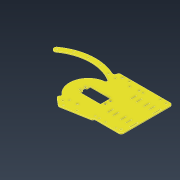
# Autodesk Inventor part: wstepna_geometria_wersja_2
Saved by Autodesk Inventor 2022 (Build 260153000, 153)
## iProperties
Created: 2022-02-09
Part Number: wstepna_geometria_wersja_2
Material: Generic
Document SubType Name: Modeling
Designer: Tomasz Krakowski
Density: 1 g/cm^3
Appearance: Kanarkowa
Mass: 25.2721 g
Surface Area: 279.808 cm^2
Volume: 25.2721 cm^3
Author: Tomasz Krakowski
Autodesk Inventor part; units mm, degrees
ref_plane "YZ Plane" through (0, 0, 0) normal (1, 0, 0) x (0, 1, 0)
ref_plane "XZ Plane" through (0, 0, 0) normal (0, 1, 0) x (-1, 0, 0)
ref_plane "XY Plane" through (0, 0, 0) normal (0, 0, 1) x (1, 0, 0)
sketch "Sketch1" plane through (0, 0, 0) normal (0, 1, 0) x (-1, 0, 0)
  arc A0 (-0.3814, 2.9757) -> (-3, 0) centre (0, 0) ccw
  line L0 (-35, 45.25) -> (5, 45.25)
  line L1 (5, 45.25) -> (5, 24.75)
  line L2 (5, 24.75) -> (-35, 24.75)
  line L3 (-35, 24.75) -> (-35, 45.25)
  line L4 (-35, 45.25) -> (5, 24.75) construction
  line L5 (5, 45.25) -> (-35, 24.75) construction
  line L6 (-5, 35) -> (-15, 35) construction
  circle A1 centre (9.25, 30) radius 2.1
  circle A2 centre (9.25, 40) radius 2.1
  line L7 (9.25, 40) -> (9.25, 30) construction
  circle A3 centre (-39.25, 40) radius 2.1
  circle A4 centre (-39.25, 30) radius 2.1
  line L8 (-39.25, 40) -> (-39.25, 30) construction
  line L9 (-39.25, 35) -> (-15, 35) construction
  line L10 (-5, 35) -> (9.25, 35) construction
  line L11 (-39.25, 40) -> (9.25, 40) construction
  line L12 (-39.25, 30) -> (9.25, 30) construction
  line L13 (-15, 35) -> (-15, 40) construction
  circle A5 centre (-5, 35) radius 10 construction
  circle A6 centre (-24.5, 35) radius 10 construction
  arc A7 (-0.3814, 2.9757) -> (0, 75) centre (-5, 39.0133) ccw
  line L14 (-105, 0) -> (0, 0) construction
  line L15 (-3, 0) -> (-105, 0) construction
  arc A8 (-3, 0) -> (-0.3814, -2.9757) centre (0, 0) ccw
  arc A9 (-1.6619, -2.4976) -> (97.0992, -0.9275) centre (46.5785, 70) ccw
  arc A10 (102.9008, -9.0725) -> (97.0992, -0.9275) centre (100, -5) ccw
  line L16 (0, 0) -> (100, 0) construction
  arc A11 (5.6849, -18.0476) -> (102.9008, -9.0725) centre (46.5785, 70) ccw
  line L17 (0, 75) -> (0, 0) construction
  line L18 (0, 0) -> (0, -15.1769) construction
  line L19 (0, 0) -> (-105, 0) construction
  line L20 (0, 75) -> (-105, 75)
  line L21 (-105, 75) -> (-105, -25)
  line L22 (0, -21.6754) -> (0, -21)
  line L23 (-4, -25) -> (-105, -25)
  arc A12 (5.6849, -18.0476) -> (0, -21.6754) centre (4, -21.6754) ccw
  arc A13 (-4, -25) -> (0, -21) centre (-4, -21) ccw
  point P0 (-5, -39.0133)
  point P1 (0, -25)
  dimension "d0" = 6
  dimension "d1" = 40
  dimension "d2" = 20.5
  dimension "d4" = 48.5
  dimension "d5" = 4.2
  dimension "d6" = 10
  dimension "d11" = 10.5
  dimension "d13" = 5
  dimension "d47" = 10
  dimension "d48" = 100
  dimension "d49" = 100
  dimension "d60" = 14.25
  dimension "d68" = 70
  dimension "d71" = 0
  dimension "d73" = 25
  dimension "d75" = 105
  dimension "d76" = 4
  dimension "d77" = 4
  dimension "d108" = 75
  dimension "d109" = 35
  dimension "d110" = 5
  constraints: 48 end point, 18 point on circle, 14 centre point, 10 tangent, 7 horizontal, 7 point on line, 5 midpoint, 5 perpendicular, 4 coincident, 4 equal radius, 3 collinear, 3 vertical, 2 parallel, 2 symmetric about line, 1 other
  measures "d0" diameter of A0
  measures "d1" distance between parallel lines of L3 L1
  measures "d2" distance between parallel lines of L0 L2
  measures "d4" distance between parallel lines of L8 L7
  measures "d5" diameter of A1
  measures "d6" distance of L7.end L7.start
  measures "d11" distance from line of L3 A6.centre
  measures "d13" horizontal distance of point (0, 0) A7.centre
  measures "d47" diameter of A10
  measures "d48" distance of L16.end point (0, 0)
  measures "d49" horizontal distance of point (0, 0) A10.centre
  measures "d60" distance from line of A5.centre L7
  measures "d68" vertical distance of point (0, 0) A9.centre
  measures "d71" distance between parallel lines of L19 L15
  measures "d73" distance from line of L23 point (0, 0)
  measures "d75" horizontal distance of point (0, 0) L20.end
  measures "d76" radius of A12
  measures "d77" radius of A13
  measures "d108" distance from line of point (0, 0) L20
  measures "d109" distance from line of L6 L14.end
  measures "d110" horizontal distance of A0.centre L6.start
extrude "Extrusion1" add sketch "Sketch1" along normal blind 2
sketch "Szkic5" plane through (0, 2, 0) normal (0, 1, 0) x (1, 0, 0)
  circle A0 centre (12.5, 20) radius 2.1
  circle A1 centre (97.5, 20) radius 2.1
  circle A2 centre (12.5, -67.5) radius 2.1
  circle A3 centre (97.5, -67.5) radius 2.1
  line L0 (12.5, 20) -> (97.5, 20) construction
  line L1 (97.5, -67.5) -> (97.5, 20) construction
  line L2 (12.5, -67.5) -> (97.5, -67.5) construction
  line L3 (0, -75) -> (105, -75) construction
  line L4 (105, -75) -> (105, 25) construction
  line L5 (105, 25) -> (4, 25) construction
  line L6 (0, 21) -> (0, 21.6754) construction
  point P0 (0, 0)
  dimension "d84" = 7.5
  dimension "d85" = 7.5
  dimension "d88" = 4.2
  dimension "d89" = 85
  dimension "d112" = 85
  dimension "d153" = 87.5
  constraints: 6 end point, 4 centre point, 3 equal radius, 2 horizontal, 1 vertical
  measures "d84" distance between parallel lines of L3 L2
  measures "d85" distance between parallel lines of L4 L1
  measures "d88" diameter of A0
  measures "d89" distance of L2.start L1.start
  measures "d112" distance of L0.start L0.end
  measures "d153" distance between parallel lines of L2 L0
extrude "Wyciągnięcie proste4" cut sketch "Szkic5" against normal up to surface (2 mm away)
sketch "Szkic6" plane through (0, 2, 0) normal (0, 1, 0) x (1, 0, 0)
  line L0 (103, -55) -> (100.9, -55)
  line L1 (100.9, -55) -> (100.9, -40)
  line L2 (100.9, -40) -> (103, -40)
  line L3 (103, -40) -> (103, -55)
  line L4 (103, -10) -> (100.9, -10)
  line L5 (100.9, -10) -> (100.9, 5)
  line L6 (100.9, 5) -> (103, 5)
  line L7 (103, 5) -> (103, -10)
  line L8 (105, 25) -> (4, 25) construction
  line L9 (100.9, -40) -> (100.9, -10) construction
  line L10 (105, -75) -> (105, 25) construction
  line L11 (100.9, -25) -> (105, -25) construction
  point P0 (0, 0)
  dimension "d92" = 15
  dimension "d94" = 30
  dimension "d168" = 2.1
  dimension "d169" = 2
  constraints: 20 end point, 4 parallel, 3 perpendicular, 2 collinear, 2 horizontal, 1 midpoint, 1 point on line, 1 vertical, 2 other
  measures "d92" distance of L4.end L5.end
  measures "d94" distance between parallel lines of L4 L2
  measures "d168" distance between parallel lines of L7 L5
extrude "Wyciągnięcie proste5" cut sketch "Szkic6" against normal up to surface (2 mm away)
sketch "Sketch7" plane through (0, 2, 0) normal (0, 1, 0) x (1, 0, 0)
  circle A0 centre (50, -70) radius 1.6
  circle A1 centre (57.5, -70) radius 1.6
  line L0 (50, -70) -> (57.5, -70) construction
  line L1 (105, -75) -> (105, 25) construction
  line L2 (0, -75) -> (105, -75) construction
  circle A2 centre (50, 15) radius 1.6
  circle A3 centre (57.5, 15) radius 1.6
  line L3 (50, 15) -> (57.5, 15) construction
  line L4 (50, 15) -> (50, -70) construction
  line L5 (57.5, 15) -> (57.5, -70) construction
  line L6 (105, 25) -> (4, 25) construction
  point P0 (0, 0)
  point P1 (105, -55)
  dimension "d98" = 3.2
  dimension "d100" = 7.5
  dimension "d101" = 5
  dimension "d104" = 3.2
  dimension "d152" = 85
  dimension "d167" = 50
  constraints: 8 end point, 4 centre point, 2 equal radius, 2 horizontal, 2 perpendicular
  measures "d98" diameter of A0
  measures "d100" distance of L0.start L0.end
  measures "d101" distance between parallel lines of L0 L2
  measures "d104" diameter of A2
  measures "d152" distance between parallel lines of L3 L0
  measures "d167" distance from line of L4 point (0, 0)
extrude "Extrusion6" cut sketch "Sketch7" against normal up to next
sketch "Sketch9" plane through (0, 0, 0) normal (0, -1, 0) x (1, 0, 0)
  line L0 (0, 75) -> (105, 75) construction
  line L1 (7.5, 75) -> (-3.7488, 88.4058)
  line L2 (-3.7488, 88.4058) -> (-20.9848, 73.9431)
  line L3 (-20.9848, 73.9431) -> (-16.3455, 68.4142)
  arc A0 (0, 75) -> (0.3814, 2.9757) centre (5, 39.0133) ccw construction
  arc A1 (0, 75) -> (-16.3455, 68.4142) centre (5, 39.0133) ccw
  line L4 (0, 75) -> (7.5, 75)
  point P0 (0, 0)
  dimension "d126" = 22.5
  dimension "d128" = 17.5
  dimension "d129" = 130
  dimension "d166" = 7.5
  constraints: 8 end point, 3 point on circle, 2 perpendicular, 1 centre point, 1 coincident, 1 horizontal, 1 point on line
  measures "d126" distance between parallel lines of L1 L3
  measures "d128" distance from line of L1.start L2
  measures "d129" angle of L0 L1
  measures "d166" horizontal distance of L1.start point (0, 0)
extrude "Extrusion7" add sketch "Sketch9" against normal up to surface (2 mm away)
sketch "Sketch8" plane through (0, 2, 0) normal (0, 1, 0) x (1, 0, 0)
  line L0 (-1.8203, -68.6056) -> (-7.6054, -75.5) construction
  line L1 (0, -75) -> (105, -75) construction
  circle A0 centre (12.5, -67.5) radius 2.1 construction
  line L2 (-7.6054, -75.5) -> (12.5, -75.5) construction
  line L3 (12.5, -75.5) -> (12.5, -67.5) construction
  line L4 (-7.6054, -75.5) -> (-12.3668, -81.1744) construction
  line L5 (-3.7488, -88.4058) -> (-20.9848, -73.9431) construction
  line L6 (-3.7488, -88.4058) -> (-20.9848, -73.9431) construction
  point P0 (0, 0)
  dimension "d114" = 9
  dimension "d115" = 50
  dimension "d132" = 22.5
  dimension "d133" = 11.25
  dimension "d134" = 8
  constraints: 8 end point, 2 coincident, 2 perpendicular, 1 horizontal, 1 midpoint
  measures "d114" distance of L0.start L0.end
  measures "d115" angle of L2 L0
  measures "d132" distance of L5.start L5.end
  measures "d133" distance of L5.start L4.end
  measures "d134" distance from line of L3.end L2
hole "Hole1" at (-1.8203, 2, 68.6056) at (-7.6054, 2, 75.5) direction (0, -1, 0) diameter 3.2 depth 7.5
sketch "Sketch11" plane through (0, 2, 0) normal (0, 1, 0) x (1, 0, 0)
  line L0 (-3.7488, -88.4058) -> (-20.9848, -73.9431) construction
  line L1 (-3.7488, -88.4058) -> (52.5, -78.4876)
  line L2 (7.5, -75) -> (105, -75) construction
  line L3 (7.5, -75) -> (-3.7488, -88.4058)
  line L4 (7.5, -75) -> (52.5, -75)
  line L5 (52.5, -78.4876) -> (52.5, -75)
  point P0 (0, 0)
  dimension "d149" = 100
  dimension "d150" = 45
  constraints: 8 end point, 1 perpendicular, 1 point on line
  measures "d149" angle of L1 L5
  measures "d150" distance from line of L2.start L5
extrude "Extrusion8" add sketch "Sketch11" against normal up to surface (2 mm away)
fillet "Fillet2" radius 3 5 edges at (52.5, 1, 75) (52.5, 1, 78.4876) (-3.7488, 1, 88.4058) (-20.9848, 1, 73.9431) (-16.3455, 1, 68.4142)
sketch "Szkic12" plane through (0, 2, 0) normal (0, 1, 0) x (1, 0, 0)
  line L0 (6, 12.5) -> (34, 12.5) construction
  circle A0 centre (6, 12.5) radius 1.5
  circle A1 centre (34, 12.5) radius 1.5
  line L1 (105, 25) -> (4, 25) construction
  point P0 (0, 0)
  dimension "d154" = 3
  dimension "d155" = 12.5
  dimension "d156" = 6
  dimension "d157" = 28
  constraints: 2 centre point, 2 coincident, 2 end point, 1 equal radius, 1 horizontal
  measures "d154" diameter of A0
  measures "d155" distance between parallel lines of L1 L0
  measures "d156" horizontal distance of L0.start point (0, 0)
  measures "d157" distance of L0.start L0.end
extrude "Wyciągnięcie proste9" cut sketch "Szkic12" against normal up to surface (2 mm away)
fillet "Fillet3" radius 5 2 edges at (105, 1, 75) (105, 1, -25)
sketch "Sketch13" plane through (0, 0, 0) normal (0, -1, 0) x (1, 0, 0)
  line L0 (-8, 32) -> (-5, 32)
  line L1 (-5, 32) -> (-5, 38)
  line L2 (-5, 38) -> (-8, 38)
  line L3 (-8, 38) -> (-8, 32)
  line L4 (-8, 32) -> (-5, 38) construction
  line L5 (-5, 32) -> (-8, 38) construction
  line L6 (-5, 24.75) -> (-5, 45.25) construction
  line L7 (-5, 45.25) -> (-5, 24.75) construction
  line L8 (-5, 35) -> (-6.5, 35) construction
  point P0 (0, 0)
  dimension "d161" = 3
  dimension "d162" = 6
  constraints: 14 end point, 3 midpoint, 2 parallel, 2 perpendicular, 1 collinear, 1 horizontal
  measures "d161" distance from line of L8.start L3
  measures "d162" distance between parallel lines of L2 L0
extrude "Extrusion10" cut sketch "Sketch13" against normal through all
fillet "Fillet4" radius 2 4 edges at (-5, 1, 32) (-5, 1, 38) (-8, 1, 32) (-8, 1, 38)
sketch "Sketch14" plane through (0, 2, 0) normal (0, 1, 0) x (1, 0, 0)
  arc A0 (1.6619, 2.4976) -> (-97.0992, 0.9275) centre (-46.5785, -70) ccw construction
  arc A1 (-102.9008, 9.0725) -> (-97.0992, 0.9275) centre (-100, 5) ccw construction
  arc A2 (13.245, 0) -> (-100, 5) centre (-46.5785, -70) ccw construction
  arc A3 (0.3814, -2.9757) -> (1.6619, 2.4976) centre (0, 0) ccw construction
  line L0 (0, 0) -> (13.245, 0) construction
  line L1 (0.6999, -82.5442) -> (45.0162, -74.7301) construction
  line L2 (-2.3711, -88.1629) -> (50.3991, -78.858) construction
  line L3 (0.6999, -82.5442) -> (1.5681, -87.4683) construction
  line L4 (70, -70) -> (90, -70) construction
  line L5 (55.5, -75) -> (100, -75) construction
  line L6 (25, 21) -> (85, 21) construction
  line L7 (100, 25) -> (4, 25) construction
  circle A4 centre (12.5, 20) radius 2.1 construction
  point P0 (-78.7683, 16.2709)
  point P1 (-78.7683, 16.2709)
  point P2 (-55.3429, 21.6626)
  point P3 (-55.3429, 21.6626)
  point P4 (-31.3202, 20.8077)
  point P5 (-31.3202, 20.8077)
  point P6 (-8.3374, 13.7643)
  point P7 (-8.3374, 13.7643)
  point P8 (22.8581, -78.6371)
  dimension "d172" = 60
  dimension "d174" = 5
  dimension "d175" = 45
  dimension "d176" = 4
  dimension "d177" = 5
  dimension "d178" = 20
  dimension "d179" = 10
  dimension "d180" = 4
  dimension "d181" = 60
  dimension "d182" = 12.5
  constraints: 10 coincident, 10 end point, 3 horizontal, 2 point on circle, 1 centre point, 1 midpoint, 13 other
  measures "d175" distance of L1.end L1.start
  measures "d176" distance from line of point (-2.371, -88.163) L3
  measures "d177" distance between parallel lines of L5 L4
  measures "d178" distance of L4.start L4.end
  measures "d179" horizontal distance of L5.end L4.end
  measures "d180" distance between parallel lines of L7 L6
  measures "d181" distance of L6.end L6.start
  measures "d182" horizontal distance of L6.start A4.centre
hole "Hole3" at (-100, 2, -5) at (-78.7683, 2, -16.2709) at (-55.3429, 2, -21.6626) at (-31.3202, 2, -20.8077) at (-8.3374, 2, -13.7643) at (25, 2, -21) at (85, 2, -21) at (0.6999, 2, 82.5442) at (22.8581, 2, 78.6371) at (70, 2, 70) at (90, 2, 70) direction (0, -1, 0) diameter 3.2 end through all
sketch "Sketch15" plane through (0, 2, 0) normal (0, 1, 0) x (1, 0, 0)
  line L0 (65.5, 4) -> (67, 4)
  line L1 (67, 4) -> (67, -7)
  line L2 (67, -7) -> (65.5, -7)
  line L3 (65.5, -7) -> (65.5, 4)
  line L4 (55, 4) -> (56.5, 4)
  line L5 (56.5, 4) -> (56.5, -7)
  line L6 (56.5, -7) -> (55, -7)
  line L7 (55, -7) -> (55, 4)
  line L8 (65.5, -41) -> (67, -41)
  line L9 (67, -41) -> (67, -52)
  line L10 (67, -52) -> (65.5, -52)
  line L11 (65.5, -52) -> (65.5, -41)
  line L12 (55, -41) -> (56.5, -41)
  line L13 (56.5, -41) -> (56.5, -52)
  line L14 (56.5, -52) -> (55, -52)
  line L15 (55, -52) -> (55, -41)
  line L16 (90.5, 4) -> (92, 4)
  line L17 (92, 4) -> (92, -7)
  line L18 (92, -7) -> (90.5, -7)
  line L19 (90.5, -7) -> (90.5, 4)
  line L20 (80, 4) -> (81.5, 4)
  line L21 (81.5, 4) -> (81.5, -7)
  line L22 (81.5, -7) -> (80, -7)
  line L23 (80, -7) -> (80, 4)
  line L24 (90.5, -41) -> (92, -41)
  line L25 (92, -41) -> (92, -52)
  line L26 (92, -52) -> (90.5, -52)
  line L27 (90.5, -52) -> (90.5, -41)
  line L28 (80, -41) -> (81.5, -41)
  line L29 (81.5, -41) -> (81.5, -52)
  line L30 (81.5, -52) -> (80, -52)
  line L31 (80, -52) -> (80, -41)
  point P0 (0, 0)
  dimension "d190" = 1.5
  dimension "d191" = 11
  dimension "d192" = 9
  dimension "d193" = 55
  dimension "d194" = 4
  dimension "d197" = 45
  dimension "d200" = 25
  constraints: 64 end point, 8 point on line, 4 parallel, 3 collinear, 3 horizontal, 2 perpendicular, 1 vertical, 46 other
  measures "d190" distance of L0.end L0.start
  measures "d191" distance of L2.end L0.start
  measures "d192" distance between parallel lines of L3 L5
  measures "d193" distance from line of L7 point (0, 0)
  measures "d194" vertical distance of L4.start point (0, 0)
  measures "d197" distance of L0.start L8.start
  measures "d200" distance of L0.start L16.start
extrude "Extrusion11" cut sketch "Sketch15" against normal through all
sketch "Sketch16" plane through (0, 2, 0) normal (0, 1, 0) x (1, 0, 0)
  line L0 (81.5, -41) -> (81.5, -52) projected
  line L1 (81.5, -52) -> (80, -52) projected
  line L2 (80, -52) -> (80, -41) projected
  line L3 (80, -41) -> (81.5, -41) projected
  line L4 (81.5, 4) -> (81.5, -7) projected
  line L5 (81.5, -7) -> (80, -7) projected
  line L6 (80, -7) -> (80, 4) projected
  line L7 (80, 4) -> (81.5, 4) projected
  line L8 (67, 4) -> (67, -7) projected
  line L9 (67, -7) -> (65.5, -7) projected
  line L10 (65.5, -7) -> (65.5, 4) projected
  line L11 (65.5, 4) -> (67, 4) projected
  line L12 (67, -41) -> (67, -52) projected
  line L13 (67, -52) -> (65.5, -52) projected
  line L14 (65.5, -52) -> (65.5, -41) projected
  line L15 (65.5, -41) -> (67, -41) projected
  line L16 (92, -41) -> (92, -52) projected
  line L17 (92, -52) -> (90.5, -52) projected
  line L18 (90.5, -52) -> (90.5, -41) projected
  line L19 (90.5, -41) -> (92, -41) projected
  line L20 (92, 4) -> (92, -7) projected
  line L21 (92, -7) -> (90.5, -7) projected
  line L22 (90.5, -7) -> (90.5, 4) projected
  line L23 (90.5, 4) -> (92, 4) projected
  line L24 (56.5, 4) -> (56.5, -7) projected
  line L25 (56.5, -7) -> (55, -7) projected
  line L26 (55, -7) -> (55, 4) projected
  line L27 (55, 4) -> (56.5, 4) projected
  line L28 (56.5, -41) -> (56.5, -52) projected
  line L29 (56.5, -52) -> (55, -52) projected
  line L30 (55, -52) -> (55, -41) projected
  line L31 (55, -41) -> (56.5, -41) projected
  circle A0 centre (70, -70) radius 1.6 projected
  circle A1 centre (0.6999, -82.5442) radius 1.6 projected
  circle A2 centre (25, 21) radius 1.6 projected
  circle A3 centre (-31.3202, 20.8077) radius 1.6 projected
  circle A4 centre (-78.7683, 16.2709) radius 1.6 projected
  circle A5 centre (-100, 5) radius 1.6 projected
  circle A6 centre (-55.3429, 21.6626) radius 1.6 projected
  circle A7 centre (-8.3374, 13.7643) radius 1.6 projected
  circle A8 centre (85, 21) radius 1.6 projected
  circle A9 centre (22.8581, -78.6371) radius 1.6 projected
  circle A10 centre (90, -70) radius 1.6 projected
  line L32 (-8, -36.127) -> (-8, -33.873) projected
  arc A11 (-6.5, -31.9365) -> (-8, -33.873) centre (-6, -33.873) ccw projected
  arc A12 (-6.5, -31.9365) -> (-5, -30) centre (-7, -30) ccw projected
  line L33 (-5, -30) -> (-5, -24.75) projected
  line L34 (-5, -24.75) -> (35, -24.75) projected
  line L35 (35, -24.75) -> (35, -45.25) projected
  line L36 (35, -45.25) -> (-5, -45.25) projected
  line L37 (-5, -45.25) -> (-5, -40) projected
  arc A13 (-5, -40) -> (-6.5, -38.0635) centre (-7, -40) ccw projected
  arc A14 (-8, -36.127) -> (-6.5, -38.0635) centre (-6, -36.127) ccw projected
  arc A15 (105, 20) -> (100, 25) centre (100, 20) ccw projected
  line L38 (100, 25) -> (4, 25) projected
  arc A16 (4, 25) -> (0, 21) centre (4, 21) ccw projected
  line L39 (0, 21) -> (0, 21.6754) projected
  arc A17 (-5.6849, 18.0476) -> (0, 21.6754) centre (-4, 21.6754) ccw projected
  arc A18 (-5.6849, 18.0476) -> (-102.9008, 9.0725) centre (-46.5785, -70) ccw projected
  arc A19 (-102.9008, 9.0725) -> (-97.0992, 0.9275) centre (-100, 5) ccw projected
  arc A20 (1.6619, 2.4976) -> (-97.0992, 0.9275) centre (-46.5785, -70) ccw projected
  arc A21 (0.3814, -2.9757) -> (1.6619, 2.4976) centre (0, 0) ccw projected
  arc A22 (0.3814, -2.9757) -> (-18.6731, -66.5747) centre (5, -39.0133) ccw projected
  arc A23 (-18.3296, -70.7788) -> (-18.6731, -66.5747) centre (-20.6278, -68.8504) ccw projected
  line L40 (-19.0564, -71.6449) -> (-18.3296, -70.7788) projected
  arc A24 (-19.0564, -71.6449) -> (-18.6866, -75.8714) centre (-16.7583, -73.5733) ccw projected
  line L41 (-4.8204, -87.5066) -> (-18.6866, -75.8714) projected
  arc A25 (-4.8204, -87.5066) -> (-2.3711, -88.1629) centre (-2.8921, -85.2084) ccw projected
  line L42 (-2.3711, -88.1629) -> (50.3991, -78.858) projected
  arc A26 (50.3991, -78.858) -> (52.6891, -76.9518) centre (49.8781, -75.9036) ccw projected
  arc A27 (55.5, -75) -> (52.6891, -76.9518) centre (55.5, -78) ccw projected
  line L43 (55.5, -75) -> (100, -75) projected
  arc A28 (100, -75) -> (105, -70) centre (100, -70) ccw projected
  line L44 (105, -70) -> (105, 20) projected
  circle A29 centre (6, 12.5) radius 1.5 projected
  circle A30 centre (34, 12.5) radius 1.5 projected
  circle A31 centre (-1.8203, -68.6056) radius 1.6 projected
  circle A32 centre (-7.6054, -75.5) radius 1.6 projected
  circle A33 centre (50, 15) radius 1.6 projected
  circle A34 centre (50, -70) radius 1.6 projected
  circle A35 centre (57.5, -70) radius 1.6 projected
  circle A36 centre (57.5, 15) radius 1.6 projected
  line L45 (103, -55) -> (100.9, -55) projected
  line L46 (100.9, -55) -> (100.9, -40) projected
  line L47 (100.9, -40) -> (103, -40) projected
  line L48 (103, -40) -> (103, -55) projected
  line L49 (100.9, -10) -> (100.9, 5) projected
  line L50 (100.9, 5) -> (103, 5) projected
  line L51 (103, 5) -> (103, -10) projected
  line L52 (103, -10) -> (100.9, -10) projected
  circle A37 centre (12.5, -67.5) radius 2.1 projected
  circle A38 centre (97.5, -67.5) radius 2.1 projected
  circle A39 centre (97.5, 20) radius 2.1 projected
  circle A40 centre (12.5, 20) radius 2.1 projected
  circle A41 centre (39.25, -30) radius 2.1 projected
  circle A42 centre (39.25, -40) radius 2.1 projected
  circle A43 centre (-9.25, -40) radius 2.1 projected
  circle A44 centre (-9.25, -30) radius 2.1 projected
  circle A45 centre (16, 7.5) radius 6
  circle A46 centre (30, 0.5) radius 6
  circle A47 centre (44, 7.5) radius 6
  line L53 (30, 0.5) -> (30, -5.5) construction
  circle A48 centre (16, -7.5) radius 6
  circle A49 centre (30, -14.5) radius 6
  circle A50 centre (44, -7.5) radius 6
  circle A51 centre (66, 12.5) radius 6
  circle A52 centre (80, 12.5) radius 6
  circle A53 centre (92.5, 12.5) radius 4
  line L54 (80, 12.5) -> (92.5, 12.5) construction
  line L55 (66, 12.5) -> (80, 12.5) construction
  circle A54 centre (54.5, -17) radius 6
  circle A55 centre (68.5, -17) radius 6
  circle A56 centre (82.5, -17) radius 6
  circle A57 centre (96.5, -17) radius 6
  circle A58 centre (54.5, -31) radius 6
  circle A59 centre (68.5, -31) radius 6
  circle A60 centre (82.5, -31) radius 6
  circle A61 centre (96.5, -31) radius 6
  line L56 (96.5, -17) -> (96.5, -31) construction
  line L57 (90.5, -41) -> (92, -41) construction
  line L58 (90.5, -7) -> (90.5, -41) construction
  line L59 (96.5, -24) -> (90.5, -24) construction
  arc A62 (0.3814, -2.9757) -> (-18.6731, -66.5747) centre (5, -39.0133) ccw construction
  circle A63 centre (5, -39.0133) radius 26.5 construction
  circle A64 centre (0.3983, -12.9159) radius 6
  circle A65 centre (-15.3002, -21.9794) radius 6
  circle A66 centre (-21.5, -39.0133) radius 6
  circle A67 centre (-15.3002, -56.0472) radius 6
  line L60 (5, -39.0133) -> (0.3983, -12.9159) construction
  line L61 (5, -39.0133) -> (31.5, -39.0133) construction
  circle A68 centre (-1.3002, -56.0472) radius 6
  line L62 (-15.3002, -56.0472) -> (-1.3002, -56.0472) construction
  circle A69 centre (12.6998, -56.0472) radius 6
  circle A70 centre (26.6998, -56.0472) radius 6
  circle A71 centre (40.6998, -56.0472) radius 6
  circle A72 centre (33.6998, -69.0472) radius 6
  line L63 (26.6998, -56.0472) -> (40.6998, -56.0472) construction
  line L64 (33.6998, -69.0472) -> (33.6998, -56.0472) construction
  circle A73 centre (54.5, -59.5) radius 6
  line L65 (54.5, -59.5) -> (54.5, -31) construction
  circle A74 centre (68.5, -59.5) radius 6
  circle A75 centre (82.5, -59.5) radius 6
  point P0 (34, -2.5)
  point P1 (30, -20.5)
  dimension "d205" = 12
  dimension "d206" = 14
  dimension "d207" = 14
  dimension "d208" = 7
  dimension "d209" = 7
  dimension "d212" = 15
  dimension "d217" = 16
  dimension "d218" = 7.5
  dimension "d219" = 12
  dimension "d222" = 14
  dimension "d227" = 12.5
  dimension "d228" = 8
  dimension "d229" = 66
  dimension "d230" = 12.5
  dimension "d233" = 14
  dimension "d236" = 14
  dimension "d239" = 6
  dimension "d242" = 120
  dimension "d244" = 53
  dimension "d245" = 100
  dimension "d246" = 14
  dimension "d249" = 14
  dimension "d254" = 13
  dimension "d256" = 28.5
  dimension "d259" = 14
  constraints: 28 centre point, 24 end point, 8 horizontal, 6 vertical, 5 equal radius, 3 midpoint, 3 perpendicular, 2 point on circle, 2 vertical alignment, 1 coincident, 1 collinear, 46 other
  measures "d205" diameter of A45
  measures "d206" horizontal distance of L53.start A45.centre
  measures "d207" horizontal distance of A47.centre L53.start
  measures "d208" vertical distance of A45.centre L53.start
  measures "d209" vertical distance of A47.centre L53.start
  measures "d212" distance of A30.centre point (34, -2.5)
  measures "d217" horizontal distance of A45.centre A21.centre
  measures "d218" vertical distance of A21.centre A45.centre
  measures "d219" diameter of A51
  measures "d222" distance of L55.start L54.start
  measures "d227" distance of L54.end L54.start
  measures "d228" diameter of A53
  measures "d229" horizontal distance of A21.centre L55.start
  measures "d230" distance from line of A21.centre L55
  measures "d233" distance of A54.centre A55.centre
  measures "d236" distance of A54.centre L65.end
  measures "d239" distance from line of L59.end L56
  measures "d244" diameter of A63
  measures "d245" angle of L61 L60
  measures "d246" distance of L62.start L62.end
  measures "d249" distance of L62.end A69.centre
  measures "d254" distance of L64.end L64.start
  measures "d256" distance of L65.end L65.start
  measures "d259" distance of L65.start A74.centre
extrude "Extrusion12" [suppressed]
equation "\"d11\" = d3"
equation "\"d3\" = 10.5"
body "Solid1"
